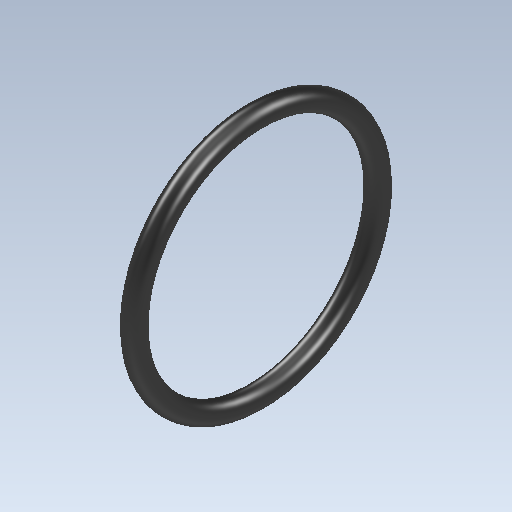
# Autodesk Inventor part: Cartridge Gland Seal M25 RS 664 4628
Saved by Autodesk Inventor 2021 (Build 250183000, 183)
## iProperties
Created: 2020-05-01
Part Number: Cartridge Gland Seal M25 RS 664 4628
Material: Generic
Document SubType Name: Modeling
Designer: jgray
Density: 1 g/cm^3
Appearance: Glossy - Black
Author: jgray
Autodesk Inventor part; units mm, degrees
ref_plane "YZ Plane" through (0, 0, 0) normal (1, 0, 0) x (0, 1, 0)
ref_plane "XZ Plane" through (0, 0, 0) normal (0, 1, 0) x (-1, 0, 0)
ref_plane "XY Plane" through (0, 0, 0) normal (0, 0, 1) x (1, 0, 0)
sketch "Sketch1" plane through (0, 0, 0) normal (0, 1, 0) x (-1, 0, 0)
  circle A0 centre (0, 0) radius 12 construction
  line L0 (12.8595, 0) -> (-16.5674, 0)
  line L1 (0, 18.0666) -> (0, -20.1794)
  circle A1 centre (0, 12) radius 1
  dimension "d0" = 24
  dimension "d1" = 2
  constraints: 4 end point, 3 point on line, 2 coincident, 1 centre point, 1 horizontal, 1 vertical, 1 vertical alignment, 2 other
  measures "d1" diameter of A1
revolve "Revolution1" add sketch "Sketch1" angle 360 about axis through (-12.8595, 0, 0) along (1, 0, 0)
body "Solid1"
